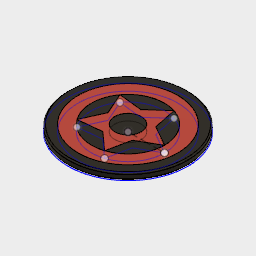
StarSaucer v1 (Autodesk Fusion 360 design; units mm, degrees)
Autodesk Fusion 360 part; units mm, degrees
sketch "Sketch1" plane through (0, 0, 0) normal (0, 1, 0) x (1, 0, 0)
  circle A0 centre (0, 0) radius 45
  circle A1 centre (0, 0) radius 37.5
  circle A2 centre (0, 0) radius 27.5
  line L0 (0, 0) -> (27.5, 0) construction
  line L1 (0, 0) -> (27.5, 0) construction
  line L2 (-22.248, -16.1641) -> (-15, 0)
  line L3 (-15, 0) -> (-22.248, 16.1641)
  line L4 (8.498, -26.1541) -> (-4.6353, -14.2658)
  line L5 (-4.6353, -14.2658) -> (-22.248, -16.1641)
  line L6 (27.5, 0) -> (12.1353, -8.8168)
  line L7 (12.1353, -8.8168) -> (8.498, -26.1541)
  line L8 (8.498, 26.1541) -> (12.1353, 8.8168)
  line L9 (12.1353, 8.8168) -> (27.5, 0)
  line L10 (-22.248, 16.1641) -> (-4.6353, 14.2658)
  line L11 (-4.6353, 14.2658) -> (8.498, 26.1541)
  circle A3 centre (0, 0) radius 10
  dimension "d2" = 90
  dimension "d3" = 75
  dimension "d12" = 360
  dimension "d13" = 20
  measures "d2" diameter of A0
  measures "d3" diameter of A1
  measures "d13" diameter of A3
extrude "Extrude1" add sketch "Sketch1" along normal blind 5 contours L2 L3 L4 L5 L6 L7 L8 L9 L10 L11 makes body 1
extrude "Extrude2" add sketch "Sketch1" along normal blind 5 separate body contours A3 makes body 2
extrude "Extrude3" add sketch "Sketch1" along normal blind 5 separate body contours A2 L8 L9 | A2 L6 L7 | A2 L10 L11 | A2 L4 L5 | A2 L2 L3 makes body 3 at (18.8409, 0, -13.6887)
extrude "Extrude4" add sketch "Sketch1" along normal blind 5 separate body contours A1 makes body 4
extrude "Extrude5" add sketch "Sketch1" along normal blind 5 separate body contours A0 makes body 5
fillet "Fillet1" radius 1 2 edges at (-41.9547, 5, 16.2727) (-41.9547, 0, 16.2727) on bodies 5
named bodies: "Star", "InnerCircle", "StarCircle", "MidCircle", "OuterCircle"
